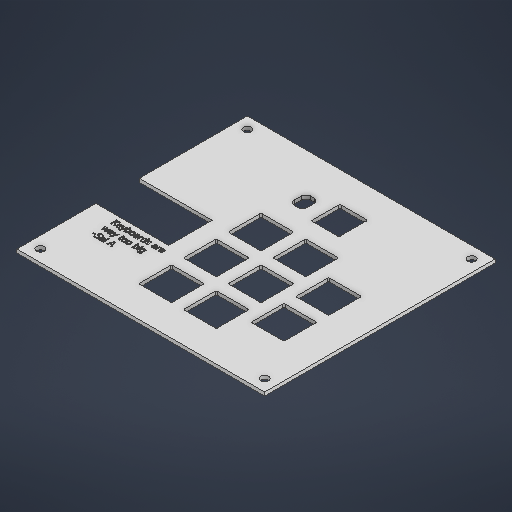
# Autodesk Inventor part: Top_Plate
Saved by Autodesk Inventor 2026 (Build 300175050, 175E)
## iProperties
Created: 2025-06-13
Part Number: Top_Plate
Material: Generic
Document SubType Name: Modeling
Designer: SaiAn
Density: 1 g/cm^3
Appearance: Default
Author: SaiAn
Autodesk Inventor part; units mm, degrees
ref_plane "YZ Plane" through (0, 0, 0) normal (1, 0, 0) x (0, 1, 0)
ref_plane "XZ Plane" through (0, 0, 0) normal (0, 1, 0) x (-1, 0, 0)
ref_plane "XY Plane" through (0, 0, 0) normal (0, 0, 1) x (1, 0, 0)
sketch "Sketch1" plane through (0, 0, 0) normal (0, 1, 0) x (-1, 0, 0)
  line L0 (0, 0) -> (105.5, 0)
  line L1 (105.5, 0) -> (105.5, -98.12)
  line L2 (105.5, -98.12) -> (0, -98.12)
  line L3 (0, -98.12) -> (0, 0)
  line L4 (34.205, -46.155) -> (47.205, -46.155)
  line L5 (33.705, -45.655) -> (33.705, -32.655)
  line L6 (47.705, -45.655) -> (47.705, -32.655)
  line L7 (34.205, -32.155) -> (47.205, -32.155)
  arc A0 (47.705, -32.655) -> (47.205, -32.155) centre (47.205, -32.655) ccw
  line L8 (34.205, -27.105) -> (47.205, -27.105)
  arc A1 (33.705, -26.605) -> (34.205, -27.105) centre (34.205, -26.605) ccw
  arc A2 (47.205, -27.105) -> (47.705, -26.605) centre (47.205, -26.605) ccw
  line L9 (33.705, -26.605) -> (33.705, -13.605)
  line L10 (47.705, -26.605) -> (47.705, -13.605)
  arc A3 (47.705, -13.605) -> (47.205, -13.105) centre (47.205, -13.605) ccw
  line L11 (34.205, -13.105) -> (47.205, -13.105)
  arc A4 (34.205, -13.105) -> (33.705, -13.605) centre (34.205, -13.605) ccw
  line L12 (33.705, -64.705) -> (33.705, -51.705)
  line L13 (47.705, -64.705) -> (47.705, -51.705)
  line L14 (34.205, -65.205) -> (47.205, -65.205)
  line L15 (34.205, -51.205) -> (47.205, -51.205)
  arc A5 (47.705, -51.705) -> (47.205, -51.205) centre (47.205, -51.705) ccw
  arc A6 (34.205, -51.205) -> (33.705, -51.705) centre (34.205, -51.705) ccw
  arc A7 (47.205, -65.205) -> (47.705, -64.705) centre (47.205, -64.705) ccw
  arc A8 (33.705, -64.705) -> (34.205, -65.205) centre (34.205, -64.705) ccw
  arc A9 (33.705, -45.655) -> (34.205, -46.155) centre (34.205, -45.655) ccw
  arc A10 (34.205, -32.155) -> (33.705, -32.655) centre (34.205, -32.655) ccw
  arc A11 (47.205, -46.155) -> (47.705, -45.655) centre (47.205, -45.655) ccw
  line L16 (52.755, -64.705) -> (52.755, -51.705)
  line L17 (66.755, -64.705) -> (66.755, -51.705)
  line L18 (53.255, -65.205) -> (66.255, -65.205)
  arc A12 (66.255, -65.205) -> (66.755, -64.705) centre (66.255, -64.705) ccw
  arc A13 (52.755, -45.655) -> (53.255, -46.155) centre (53.255, -45.655) ccw
  arc A14 (53.255, -51.205) -> (52.755, -51.705) centre (53.255, -51.705) ccw
  arc A15 (66.255, -46.155) -> (66.755, -45.655) centre (66.255, -45.655) ccw
  line L19 (53.255, -51.205) -> (66.255, -51.205)
  arc A16 (52.755, -64.705) -> (53.255, -65.205) centre (53.255, -64.705) ccw
  line L20 (53.255, -46.155) -> (66.255, -46.155)
  line L21 (66.755, -45.655) -> (66.755, -32.655)
  line L22 (53.255, -32.155) -> (66.255, -32.155)
  arc A17 (53.255, -32.155) -> (52.755, -32.655) centre (53.255, -32.655) ccw
  line L23 (52.755, -45.655) -> (52.755, -32.655)
  arc A18 (66.755, -51.705) -> (66.255, -51.205) centre (66.255, -51.705) ccw
  arc A19 (66.755, -32.655) -> (66.255, -32.155) centre (66.255, -32.655) ccw
  line L24 (53.255, -27.105) -> (66.255, -27.105)
  arc A20 (52.755, -26.605) -> (53.255, -27.105) centre (53.255, -26.605) ccw
  arc A21 (66.255, -27.105) -> (66.755, -26.605) centre (66.255, -26.605) ccw
  line L25 (52.755, -26.605) -> (52.755, -13.605)
  line L26 (53.255, -13.105) -> (66.255, -13.105)
  line L27 (66.755, -26.605) -> (66.755, -13.605)
  arc A22 (53.255, -13.105) -> (52.755, -13.605) centre (53.255, -13.605) ccw
  arc A23 (66.755, -13.605) -> (66.255, -13.105) centre (66.255, -13.605) ccw
  line L28 (14.6002, -55.3601) -> (14.6002, -42.3601)
  arc A24 (14.6002, -55.3601) -> (15.1002, -55.8601) centre (15.1002, -55.3601) ccw
  arc A25 (28.6002, -42.3601) -> (28.1002, -41.8601) centre (28.1002, -42.3601) ccw
  arc A26 (28.1002, -55.8601) -> (28.6002, -55.3601) centre (28.1002, -55.3601) ccw
  line L29 (28.6002, -55.3601) -> (28.6002, -42.3601)
  line L30 (15.1002, -55.8601) -> (28.1002, -55.8601)
  line L31 (15.1002, -41.8601) -> (28.1002, -41.8601)
  arc A27 (15.1002, -41.8601) -> (14.6002, -42.3601) centre (15.1002, -42.3601) ccw
  line L32 (15.1002, -36.8101) -> (28.1002, -36.8101)
  arc A28 (28.1002, -36.8101) -> (28.6002, -36.3101) centre (28.1002, -36.3101) ccw
  line L33 (14.6002, -36.3101) -> (14.6002, -23.3101)
  line L34 (28.6002, -36.3101) -> (28.6002, -23.3101)
  arc A29 (15.1002, -22.8101) -> (14.6002, -23.3101) centre (15.1002, -23.3101) ccw
  line L35 (15.1002, -22.8101) -> (28.1002, -22.8101)
  arc A30 (28.6002, -23.3101) -> (28.1002, -22.8101) centre (28.1002, -23.3101) ccw
  arc A31 (14.6002, -36.3101) -> (15.1002, -36.8101) centre (15.1002, -36.3101) ccw
  line L36 (62.477, -82.084) -> (60.977, -82.084)
  line L37 (58.977, -80.084) -> (58.977, -77.084)
  line L38 (60.977, -75.084) -> (62.477, -75.084)
  line L39 (64.477, -77.084) -> (64.477, -80.084)
  arc A32 (64.477, -77.084) -> (62.477, -75.084) centre (62.477, -77.084) ccw
  arc A33 (62.477, -82.084) -> (64.477, -80.084) centre (62.477, -80.084) ccw
  arc A34 (60.977, -75.084) -> (58.977, -77.084) centre (60.977, -77.084) ccw
  arc A35 (58.977, -80.084) -> (60.977, -82.084) centre (60.977, -80.084) ccw
  line L40 (105.5, -98.12) -> (105.5, -85.262)
  line L41 (52.74, -85.262) -> (41.94, -85.262)
  line L42 (41.44, -84.762) -> (41.44, -73.562)
  line L43 (41.94, -73.062) -> (52.74, -73.062)
  line L44 (53.24, -73.562) -> (53.24, -84.762)
  arc A36 (52.74, -85.262) -> (53.24, -84.762) centre (52.74, -84.762) ccw
  arc A37 (53.24, -73.562) -> (52.74, -73.062) centre (52.74, -73.562) ccw
  arc A38 (41.94, -73.062) -> (41.44, -73.562) centre (41.94, -73.562) ccw
  arc A39 (41.44, -84.762) -> (41.94, -85.262) centre (41.94, -84.762) ccw
  line L45 (105.5, -33.622) -> (74.5, -33.622)
  line L46 (74.5, -33.622) -> (74.5, -52.122)
  line L47 (74.5, -52.122) -> (105.5, -52.122)
  line L48 (105.5, -33.622) -> (105.5, -52.122)
  circle A40 centre (100.5, -5) radius 1.7
  circle A41 centre (100.5, -93.12) radius 1.7
  circle A42 centre (5, -5) radius 1.7
  circle A43 centre (5, -93.12) radius 1.7
  point P0 (53.24, -85.262)
  point P1 (41.44, -73.062)
  point P2 (41.44, -85.262)
  point P3 (53.24, -73.062)
  point P4 (15.1002, -22.8101)
  point P5 (28.6002, -36.3101)
  point P6 (15.1002, -55.8601)
  point P7 (28.1002, -41.8601)
  point P8 (28.6002, -42.3601)
  point P9 (28.6002, -55.3601)
  point P10 (28.1002, -55.8601)
  point P11 (66.755, -26.605)
  point P12 (66.755, -45.655)
  point P13 (66.255, -46.155)
  point P14 (53.255, -46.155)
  point P15 (52.755, -45.655)
  point P16 (52.755, -32.655)
  point P17 (53.255, -51.205)
  point P18 (33.705, -26.605)
  point P19 (47.205, -13.105)
  point P20 (47.705, -26.605)
  dimension "d0" = 105.5
  dimension "d1" = 98.12
  dimension "d16" = 2
  dimension "d17" = 2
  dimension "d18" = 2
  dimension "d19" = 2
  dimension "d21" = 52.26
  dimension "d22" = 11.8
  dimension "d23" = 12.2
  dimension "d24" = 0.5
  dimension "d26" = 31
  dimension "d28" = 18.5
  dimension "d29" = 3.4
  dimension "d30" = 3.4
  dimension "d31" = 3.4
  dimension "d32" = 3.4
  dimension "d33" = 5
  dimension "d34" = 5
  dimension "d35" = 5
  dimension "d36" = 5
  dimension "d37" = 5
  dimension "d38" = 5
  dimension "d39" = 5
  dimension "d40" = 5
  constraints: 98 end point, 80 point on circle, 44 centre point, 16 tangent, 11 point on line, 6 parallel, 5 perpendicular, 3 equal radius, 3 horizontal, 1 collinear
  measures "d0" distance of L1.end L2.end
  measures "d1" distance of L0.end L1.end
  measures "d16" radius of A32
  measures "d17" radius of A33
  measures "d18" radius of A34
  measures "d19" radius of A35
  measures "d21" distance of L40.end point (53.24, -85.262)
  measures "d22" distance of point (41.44, -73.062) point (53.24, -73.062)
  measures "d23" distance of point (41.44, -85.262) point (41.44, -73.062)
  measures "d24" radius of A36
  measures "d26" distance of L45.start L45.end
  measures "d28" distance of L45.end L46.end
  measures "d29" diameter of A40
  measures "d30" diameter of A41
  measures "d31" diameter of A42
  measures "d32" diameter of A43
  measures "d33" distance from line of L1 A40.centre
  measures "d34" distance from line of L0 A40.centre
  measures "d35" distance from line of L2 A41.centre
  measures "d36" distance from line of L1 A41.centre
  measures "d37" distance from line of L0 A42.centre
  measures "d38" distance from line of L3 A42.centre
  measures "d39" distance from line of L2 A43.centre
  measures "d40" distance from line of L3 A43.centre
extrude "Extrusion1" add sketch "Sketch1" along normal blind 1.5 contours L0 L1 L45 L46 L47 L2 L3
sketch "Sketch3" plane through (0, 1.5, 0) normal (0, 1, 0) x (1, 0, 0)
  line L0 (-95.2585, 32.0285) -> (-71.0604, 32.0285) construction
  line L1 (-71.0604, 32.0285) -> (-71.0604, 1.6863) construction
  line L2 (-71.0604, 1.6863) -> (-95.2585, 1.6863) construction
  line L3 (-95.2585, 1.6863) -> (-95.2585, 32.0285) construction
  line L4 (-93.1487, 29.3753) -> (-93.5871, 29.3753)
  line L5 (-93.5871, 29.3753) -> (-94.5154, 30.5567)
  line L6 (-94.5154, 30.5567) -> (-94.6636, 30.39)
  line L7 (-94.6636, 30.39) -> (-94.6636, 29.3753)
  line L8 (-94.6636, 29.3753) -> (-95.0012, 29.3753)
  line L9 (-95.0012, 29.3753) -> (-95.0012, 31.9153)
  line L10 (-95.0012, 31.9153) -> (-94.6636, 31.9153)
  line L11 (-94.6636, 31.9153) -> (-94.6636, 30.7482)
  line L12 (-94.6636, 30.7482) -> (-93.6221, 31.9153)
  line L13 (-93.6221, 31.9153) -> (-93.2104, 31.9153)
  line L14 (-93.2104, 31.9153) -> (-94.2623, 30.7811)
  line L15 (-94.2623, 30.7811) -> (-93.1487, 29.3753)
  spline S0 degree 2 poles (-92.1442, 29.332) (-92.6012, 29.332) (-93.1034, 29.8446) (-93.1034, 30.318) knots 0 0 0 1 2 2 2
  spline S1 degree 2 poles (-93.1034, 30.318) (-93.1034, 30.7832) (-92.6156, 31.3348) (-92.2224, 31.3348) knots 0 0 0 1 2 2 2
  spline S2 degree 2 poles (-92.2224, 31.3348) (-92.0454, 31.3348) (-91.7717, 31.2319) (-91.6708, 31.1228) knots 0 0 0 1 2 2 2
  spline S3 degree 2 poles (-91.6708, 31.1228) (-91.5679, 31.0137) (-91.4588, 30.6988) (-91.4588, 30.4703) knots 0 0 0 1 2 2 2
  line L16 (-91.4588, 30.4703) -> (-91.4588, 30.2953)
  line L17 (-91.4588, 30.2953) -> (-92.7782, 30.2953)
  spline S4 degree 2 poles (-92.7782, 30.2953) (-92.7782, 29.9639) (-92.4447, 29.612) (-92.1483, 29.612) knots 0 0 0 1 2 2 2
  spline S5 degree 2 poles (-92.1483, 29.612) (-92.0434, 29.612) (-91.8396, 29.6593) (-91.7572, 29.6964) knots 0 0 0 1 2 2 2
  spline S6 degree 2 poles (-91.7572, 29.6964) (-91.6708, 29.7375) (-91.5514, 29.8096) (-91.5123, 29.8425) knots 0 0 0 1 2 2 2
  line L18 (-91.5123, 29.8425) -> (-91.4938, 29.8425)
  line L19 (-91.4938, 29.8425) -> (-91.4938, 29.4926)
  spline S7 degree 2 poles (-91.4938, 29.4926) (-91.5494, 29.4699) (-91.7181, 29.4041) (-91.784, 29.3855) knots 0 0 0 1 2 2 2
  spline S8 degree 2 poles (-91.784, 29.3855) (-91.8766, 29.3588) (-92.0289, 29.332) (-92.1442, 29.332) knots 0 0 0 1 2 2 2
  spline S9 degree 2 poles (-91.7717, 30.5403) (-91.7758, 30.67) (-91.8293, 30.8593) (-91.8807, 30.9231) knots 0 0 0 1 2 2 2
  spline S10 degree 2 poles (-91.8807, 30.9231) (-91.9363, 30.9952) (-92.1113, 31.0713) (-92.241, 31.0713) knots 0 0 0 1 2 2 2
  spline S11 degree 2 poles (-92.241, 31.0713) (-92.3686, 31.0713) (-92.5476, 30.9952) (-92.6217, 30.9211) knots 0 0 0 1 2 2 2
  spline S12 degree 2 poles (-92.6217, 30.9211) (-92.6938, 30.8449) (-92.7679, 30.6617) (-92.7782, 30.5403) knots 0 0 0 1 2 2 2
  line L20 (-92.7782, 30.5403) -> (-91.7717, 30.5403)
  line L21 (-89.6371, 31.2813) -> (-90.6622, 28.6734)
  line L22 (-90.6622, 28.6734) -> (-91.0059, 28.6734)
  line L23 (-91.0059, 28.6734) -> (-90.6643, 29.4679)
  line L24 (-90.6643, 29.4679) -> (-91.3559, 31.2813)
  line L25 (-91.3559, 31.2813) -> (-91.0101, 31.2813)
  line L26 (-91.0101, 31.2813) -> (-90.4893, 29.8693)
  line L27 (-90.4893, 29.8693) -> (-89.9706, 31.2813)
  line L28 (-89.9706, 31.2813) -> (-89.6371, 31.2813)
  spline S13 degree 2 poles (-87.797, 30.3591) (-87.797, 29.8919) (-88.2498, 29.3217) (-88.5915, 29.3217) knots 0 0 0 1 2 2 2
  spline S14 degree 2 poles (-88.5915, 29.3217) (-88.7459, 29.3217) (-88.9661, 29.3979) (-89.0732, 29.4638) knots 0 0 0 1 2 2 2
  line L29 (-89.0732, 29.4638) -> (-89.0937, 29.3753)
  line L30 (-89.0937, 29.3753) -> (-89.3943, 29.3753)
  line L31 (-89.3943, 29.3753) -> (-89.3943, 32.0285)
  line L32 (-89.3943, 32.0285) -> (-89.0732, 32.0285)
  line L33 (-89.0732, 32.0285) -> (-89.0732, 31.0816)
  spline S15 degree 2 poles (-89.0732, 31.0816) (-88.9517, 31.1907) (-88.6697, 31.3348) (-88.4906, 31.3348) knots 0 0 0 1 2 2 2
  spline S16 degree 2 poles (-88.4906, 31.3348) (-88.1675, 31.3348) (-87.797, 30.8182) (-87.797, 30.3591) knots 0 0 0 1 2 2 2
  spline S17 degree 2 poles (-88.1284, 30.3344) (-88.1284, 30.6761) (-88.3363, 31.0302) (-88.5668, 31.0302) knots 0 0 0 1 2 2 2
  spline S18 degree 2 poles (-88.5668, 31.0302) (-88.6965, 31.0302) (-88.9641, 30.9067) (-89.0732, 30.812) knots 0 0 0 1 2 2 2
  line L34 (-89.0732, 30.812) -> (-89.0732, 29.719)
  spline S19 degree 2 poles (-89.0732, 29.719) (-88.9517, 29.6593) (-88.7644, 29.6099) (-88.6533, 29.6099) knots 0 0 0 1 2 2 2
  spline S20 degree 2 poles (-88.6533, 29.6099) (-88.4083, 29.6099) (-88.1284, 29.9578) (-88.1284, 30.3344) knots 0 0 0 1 2 2 2
  spline S21 degree 2 poles (-85.8971, 30.3283) (-85.8971, 29.8466) (-86.3603, 29.3217) (-86.7472, 29.3217) knots 0 0 0 1 2 2 2
  spline S22 degree 2 poles (-86.7472, 29.3217) (-87.1445, 29.3217) (-87.5994, 29.8631) (-87.5994, 30.3283) knots 0 0 0 1 2 2 2
  spline S23 degree 2 poles (-87.5994, 30.3283) (-87.5994, 30.8058) (-87.1301, 31.3348) (-86.7472, 31.3348) knots 0 0 0 1 2 2 2
  spline S24 degree 2 poles (-86.7472, 31.3348) (-86.3603, 31.3348) (-85.8971, 30.8079) (-85.8971, 30.3283) knots 0 0 0 1 2 2 2
  spline S25 degree 2 poles (-86.2285, 30.3283) (-86.2285, 30.6988) (-86.4982, 31.059) (-86.7472, 31.059) knots 0 0 0 1 2 2 2
  spline S26 degree 2 poles (-86.7472, 31.059) (-86.9963, 31.059) (-87.268, 30.6988) (-87.268, 30.3283) knots 0 0 0 1 2 2 2
  spline S27 degree 2 poles (-87.268, 30.3283) (-87.268, 29.9681) (-86.9963, 29.5976) (-86.7472, 29.5976) knots 0 0 0 1 2 2 2
  spline S28 degree 2 poles (-86.7472, 29.5976) (-86.5002, 29.5976) (-86.2285, 29.9619) (-86.2285, 30.3283) knots 0 0 0 1 2 2 2
  spline S29 degree 2 poles (-84.5057, 29.577) (-84.5448, 29.5482) (-84.6765, 29.4452) (-84.7383, 29.4144) knots 0 0 0 1 2 2 2
  spline S30 degree 2 poles (-84.7383, 29.4144) (-84.8227, 29.3691) (-84.9812, 29.3217) (-85.1252, 29.3217) knots 0 0 0 1 2 2 2
  spline S31 degree 2 poles (-85.1252, 29.3217) (-85.2426, 29.3217) (-85.4546, 29.4102) (-85.5349, 29.4905) knots 0 0 0 1 2 2 2
  spline S32 degree 2 poles (-85.5349, 29.4905) (-85.611, 29.5687) (-85.7036, 29.7993) (-85.7036, 29.9269) knots 0 0 0 1 2 2 2
  spline S33 degree 2 poles (-85.7036, 29.9269) (-85.7036, 30.1245) (-85.5369, 30.4044) (-85.3558, 30.4847) knots 0 0 0 1 2 2 2
  spline S34 degree 2 poles (-85.3558, 30.4847) (-85.1952, 30.5588) (-84.7589, 30.6144) (-84.5057, 30.6288) knots 0 0 0 1 2 2 2
  line L35 (-84.5057, 30.6288) -> (-84.5057, 30.6905)
  spline S35 degree 2 poles (-84.5057, 30.6905) (-84.5057, 30.8017) (-84.5736, 30.9396) (-84.6354, 30.9787) knots 0 0 0 1 2 2 2
  spline S36 degree 2 poles (-84.6354, 30.9787) (-84.6971, 31.0178) (-84.8741, 31.0425) (-84.9688, 31.0425) knots 0 0 0 1 2 2 2
  spline S37 degree 2 poles (-84.9688, 31.0425) (-85.08, 31.0425) (-85.3805, 30.9766) (-85.5307, 30.9128) knots 0 0 0 1 2 2 2
  line L36 (-85.5307, 30.9128) -> (-85.5493, 30.9128)
  line L37 (-85.5493, 30.9128) -> (-85.5493, 31.2401)
  spline S38 degree 2 poles (-85.5493, 31.2401) (-85.4608, 31.2648) (-85.1294, 31.3266) (-84.9668, 31.3266) knots 0 0 0 1 2 2 2
  spline S39 degree 2 poles (-84.9668, 31.3266) (-84.7692, 31.3266) (-84.4995, 31.2648) (-84.3925, 31.1845) knots 0 0 0 1 2 2 2
  spline S40 degree 2 poles (-84.3925, 31.1845) (-84.2875, 31.1063) (-84.1846, 30.8573) (-84.1846, 30.6782) knots 0 0 0 1 2 2 2
  line L38 (-84.1846, 30.6782) -> (-84.1846, 29.3753)
  line L39 (-84.1846, 29.3753) -> (-84.5057, 29.3753)
  line L40 (-84.5057, 29.3753) -> (-84.5057, 29.577)
  line L41 (-84.5057, 29.8446) -> (-84.5057, 30.3736)
  spline S41 degree 2 poles (-84.5057, 30.3736) (-84.621, 30.3633) (-84.9688, 30.3283) (-85.0779, 30.2953) knots 0 0 0 1 2 2 2
  spline S42 degree 2 poles (-85.0779, 30.2953) (-85.2055, 30.2562) (-85.3723, 30.0936) (-85.3723, 29.9495) knots 0 0 0 1 2 2 2
  spline S43 degree 2 poles (-85.3723, 29.9495) (-85.3723, 29.7849) (-85.187, 29.6181) (-85.01, 29.6181) knots 0 0 0 1 2 2 2
  spline S44 degree 2 poles (-85.01, 29.6181) (-84.8597, 29.6181) (-84.6127, 29.7478) (-84.5057, 29.8446) knots 0 0 0 1 2 2 2
  line L42 (-82.7232, 30.9375) -> (-82.7396, 30.9375)
  spline S45 degree 2 poles (-82.7396, 30.9375) (-82.7767, 30.9478) (-82.857, 30.9519) (-82.9125, 30.9519) knots 0 0 0 1 2 2 2
  spline S46 degree 2 poles (-82.9125, 30.9519) (-83.0422, 30.9519) (-83.2974, 30.8387) (-83.4127, 30.7276) knots 0 0 0 1 2 2 2
  line L43 (-83.4127, 30.7276) -> (-83.4127, 29.3753)
  line L44 (-83.4127, 29.3753) -> (-83.7338, 29.3753)
  line L45 (-83.7338, 29.3753) -> (-83.7338, 31.2813)
  line L46 (-83.7338, 31.2813) -> (-83.4127, 31.2813)
  line L47 (-83.4127, 31.2813) -> (-83.4127, 30.9972)
  spline S47 degree 2 poles (-83.4127, 30.9972) (-83.2377, 31.1537) (-82.9763, 31.2813) (-82.8528, 31.2813) knots 0 0 0 1 2 2 2
  spline S48 degree 2 poles (-82.8528, 31.2813) (-82.8034, 31.2813) (-82.754, 31.2772) (-82.7232, 31.271) knots 0 0 0 1 2 2 2
  line L48 (-82.7232, 31.271) -> (-82.7232, 30.9375)
  line L49 (-81.0086, 29.3753) -> (-81.3297, 29.3753)
  line L50 (-81.3297, 29.3753) -> (-81.3297, 29.5687)
  spline S49 degree 2 poles (-81.3297, 29.5687) (-81.4038, 29.507) (-81.5129, 29.4247) (-81.587, 29.3897) knots 0 0 0 1 2 2 2
  spline S50 degree 2 poles (-81.587, 29.3897) (-81.6549, 29.3567) (-81.801, 29.3217) (-81.8978, 29.3217) knots 0 0 0 1 2 2 2
  spline S51 degree 2 poles (-81.8978, 29.3217) (-82.0542, 29.3217) (-82.3177, 29.4514) (-82.4103, 29.577) knots 0 0 0 1 2 2 2
  spline S52 degree 2 poles (-82.4103, 29.577) (-82.5029, 29.7025) (-82.6058, 30.073) (-82.6058, 30.3139) knots 0 0 0 1 2 2 2
  spline S53 degree 2 poles (-82.6058, 30.3139) (-82.6058, 30.565) (-82.4762, 30.9314) (-82.3629, 31.0693) knots 0 0 0 1 2 2 2
  spline S54 degree 2 poles (-82.3629, 31.0693) (-82.258, 31.1928) (-81.9636, 31.3348) (-81.801, 31.3348) knots 0 0 0 1 2 2 2
  spline S55 degree 2 poles (-81.801, 31.3348) (-81.659, 31.3348) (-81.447, 31.271) (-81.3297, 31.2051) knots 0 0 0 1 2 2 2
  line L51 (-81.3297, 31.2051) -> (-81.3297, 32.0285)
  line L52 (-81.3297, 32.0285) -> (-81.0086, 32.0285)
  line L53 (-81.0086, 32.0285) -> (-81.0086, 29.3753)
  line L54 (-81.3297, 29.8384) -> (-81.3297, 30.9396)
  spline S56 degree 2 poles (-81.3297, 30.9396) (-81.449, 30.9972) (-81.6384, 31.0405) (-81.7475, 31.0405) knots 0 0 0 1 2 2 2
  spline S57 degree 2 poles (-81.7475, 31.0405) (-81.9945, 31.0405) (-82.2744, 30.67) (-82.2744, 30.32) knots 0 0 0 1 2 2 2
  spline S58 degree 2 poles (-82.2744, 30.32) (-82.2744, 29.9825) (-82.0604, 29.6264) (-81.8237, 29.6264) knots 0 0 0 1 2 2 2
  spline S59 degree 2 poles (-81.8237, 29.6264) (-81.6981, 29.6264) (-81.4429, 29.7416) (-81.3297, 29.8384) knots 0 0 0 1 2 2 2
  spline S60 degree 2 poles (-80.0288, 29.33) (-80.2202, 29.33) (-80.5516, 29.4329) (-80.6607, 29.4905) knots 0 0 0 1 2 2 2
  line L55 (-80.6607, 29.4905) -> (-80.6607, 29.8507)
  line L56 (-80.6607, 29.8507) -> (-80.6442, 29.8507)
  spline S61 degree 2 poles (-80.6442, 29.8507) (-80.6031, 29.8178) (-80.4919, 29.7396) (-80.3993, 29.6964) knots 0 0 0 1 2 2 2
  spline S62 degree 2 poles (-80.3993, 29.6964) (-80.319, 29.6572) (-80.1214, 29.5996) (-80.0164, 29.5996) knots 0 0 0 1 2 2 2
  spline S63 degree 2 poles (-80.0164, 29.5996) (-79.9403, 29.5996) (-79.7653, 29.6346) (-79.7241, 29.6634) knots 0 0 0 1 2 2 2
  spline S64 degree 2 poles (-79.7241, 29.6634) (-79.6645, 29.7025) (-79.6109, 29.791) (-79.6109, 29.8816) knots 0 0 0 1 2 2 2
  spline S65 degree 2 poles (-79.6109, 29.8816) (-79.6109, 29.9948) (-79.7344, 30.1121) (-79.8929, 30.1513) knots 0 0 0 1 2 2 2
  spline S66 degree 2 poles (-79.8929, 30.1513) (-79.9547, 30.1657) (-80.1523, 30.2068) (-80.2367, 30.2295) knots 0 0 0 1 2 2 2
  spline S67 degree 2 poles (-80.2367, 30.2295) (-80.4549, 30.2933) (-80.6525, 30.5567) (-80.6525, 30.7441) knots 0 0 0 1 2 2 2
  spline S68 degree 2 poles (-80.6525, 30.7441) (-80.6525, 31.0034) (-80.2634, 31.3266) (-79.9423, 31.3266) knots 0 0 0 1 2 2 2
  spline S69 degree 2 poles (-79.9423, 31.3266) (-79.7838, 31.3266) (-79.4627, 31.2483) (-79.3536, 31.1887) knots 0 0 0 1 2 2 2
  line L57 (-79.3536, 31.1887) -> (-79.3536, 30.8449)
  line L58 (-79.3536, 30.8449) -> (-79.3701, 30.8449)
  spline S70 degree 2 poles (-79.3701, 30.8449) (-79.4936, 30.9437) (-79.7941, 31.0569) (-79.9485, 31.0569) knots 0 0 0 1 2 2 2
  spline S71 degree 2 poles (-79.9485, 31.0569) (-80.107, 31.0569) (-80.3252, 30.9231) (-80.3252, 30.7893) knots 0 0 0 1 2 2 2
  spline S72 degree 2 poles (-80.3252, 30.7893) (-80.3252, 30.6679) (-80.1955, 30.5506) (-80.0514, 30.5135) knots 0 0 0 1 2 2 2
  spline S73 degree 2 poles (-80.0514, 30.5135) (-79.9814, 30.495) (-79.8044, 30.4579) (-79.7077, 30.4353) knots 0 0 0 1 2 2 2
  spline S74 degree 2 poles (-79.7077, 30.4353) (-79.4977, 30.3818) (-79.2837, 30.1368) (-79.2837, 29.9248) knots 0 0 0 1 2 2 2
  spline S75 degree 2 poles (-79.2837, 29.9248) (-79.2837, 29.8013) (-79.3804, 29.5831) (-79.4751, 29.5029) knots 0 0 0 1 2 2 2
  spline S76 degree 2 poles (-79.4751, 29.5029) (-79.5759, 29.4185) (-79.8332, 29.33) (-80.0288, 29.33) knots 0 0 0 1 2 2 2
  spline S77 degree 2 poles (-76.8322, 29.577) (-76.8713, 29.5482) (-77.003, 29.4452) (-77.0648, 29.4144) knots 0 0 0 1 2 2 2
  spline S78 degree 2 poles (-77.0648, 29.4144) (-77.1492, 29.3691) (-77.3076, 29.3217) (-77.4517, 29.3217) knots 0 0 0 1 2 2 2
  spline S79 degree 2 poles (-77.4517, 29.3217) (-77.5691, 29.3217) (-77.7811, 29.4102) (-77.8613, 29.4905) knots 0 0 0 1 2 2 2
  spline S80 degree 2 poles (-77.8613, 29.4905) (-77.9375, 29.5687) (-78.0301, 29.7993) (-78.0301, 29.9269) knots 0 0 0 1 2 2 2
  spline S81 degree 2 poles (-78.0301, 29.9269) (-78.0301, 30.1245) (-77.8634, 30.4044) (-77.6823, 30.4847) knots 0 0 0 1 2 2 2
  spline S82 degree 2 poles (-77.6823, 30.4847) (-77.5217, 30.5588) (-77.0853, 30.6144) (-76.8322, 30.6288) knots 0 0 0 1 2 2 2
  line L59 (-76.8322, 30.6288) -> (-76.8322, 30.6905)
  spline S83 degree 2 poles (-76.8322, 30.6905) (-76.8322, 30.8017) (-76.9001, 30.9396) (-76.9618, 30.9787) knots 0 0 0 1 2 2 2
  spline S84 degree 2 poles (-76.9618, 30.9787) (-77.0236, 31.0178) (-77.2006, 31.0425) (-77.2953, 31.0425) knots 0 0 0 1 2 2 2
  spline S85 degree 2 poles (-77.2953, 31.0425) (-77.4064, 31.0425) (-77.707, 30.9766) (-77.8572, 30.9128) knots 0 0 0 1 2 2 2
  line L60 (-77.8572, 30.9128) -> (-77.8758, 30.9128)
  line L61 (-77.8758, 30.9128) -> (-77.8758, 31.2401)
  spline S86 degree 2 poles (-77.8758, 31.2401) (-77.7872, 31.2648) (-77.4558, 31.3266) (-77.2932, 31.3266) knots 0 0 0 1 2 2 2
  spline S87 degree 2 poles (-77.2932, 31.3266) (-77.0956, 31.3266) (-76.826, 31.2648) (-76.719, 31.1845) knots 0 0 0 1 2 2 2
  spline S88 degree 2 poles (-76.719, 31.1845) (-76.614, 31.1063) (-76.5111, 30.8573) (-76.5111, 30.6782) knots 0 0 0 1 2 2 2
  line L62 (-76.5111, 30.6782) -> (-76.5111, 29.3753)
  line L63 (-76.5111, 29.3753) -> (-76.8322, 29.3753)
  line L64 (-76.8322, 29.3753) -> (-76.8322, 29.577)
  line L65 (-76.8322, 29.8446) -> (-76.8322, 30.3736)
  spline S89 degree 2 poles (-76.8322, 30.3736) (-76.9474, 30.3633) (-77.2953, 30.3283) (-77.4044, 30.2953) knots 0 0 0 1 2 2 2
  spline S90 degree 2 poles (-77.4044, 30.2953) (-77.532, 30.2562) (-77.6987, 30.0936) (-77.6987, 29.9495) knots 0 0 0 1 2 2 2
  spline S91 degree 2 poles (-77.6987, 29.9495) (-77.6987, 29.7849) (-77.5135, 29.6181) (-77.3365, 29.6181) knots 0 0 0 1 2 2 2
  spline S92 degree 2 poles (-77.3365, 29.6181) (-77.1862, 29.6181) (-76.9392, 29.7478) (-76.8322, 29.8446) knots 0 0 0 1 2 2 2
  line L66 (-75.0496, 30.9375) -> (-75.0661, 30.9375)
  spline S93 degree 2 poles (-75.0661, 30.9375) (-75.1032, 30.9478) (-75.1834, 30.9519) (-75.239, 30.9519) knots 0 0 0 1 2 2 2
  spline S94 degree 2 poles (-75.239, 30.9519) (-75.3687, 30.9519) (-75.6239, 30.8387) (-75.7392, 30.7276) knots 0 0 0 1 2 2 2
  line L67 (-75.7392, 30.7276) -> (-75.7392, 29.3753)
  line L68 (-75.7392, 29.3753) -> (-76.0603, 29.3753)
  line L69 (-76.0603, 29.3753) -> (-76.0603, 31.2813)
  line L70 (-76.0603, 31.2813) -> (-75.7392, 31.2813)
  line L71 (-75.7392, 31.2813) -> (-75.7392, 30.9972)
  spline S95 degree 2 poles (-75.7392, 30.9972) (-75.5642, 31.1537) (-75.3028, 31.2813) (-75.1793, 31.2813) knots 0 0 0 1 2 2 2
  spline S96 degree 2 poles (-75.1793, 31.2813) (-75.1299, 31.2813) (-75.0805, 31.2772) (-75.0496, 31.271) knots 0 0 0 1 2 2 2
  line L72 (-75.0496, 31.271) -> (-75.0496, 30.9375)
  spline S97 degree 2 poles (-73.9731, 29.332) (-74.4301, 29.332) (-74.9323, 29.8446) (-74.9323, 30.318) knots 0 0 0 1 2 2 2
  spline S98 degree 2 poles (-74.9323, 30.318) (-74.9323, 30.7832) (-74.4445, 31.3348) (-74.0513, 31.3348) knots 0 0 0 1 2 2 2
  spline S99 degree 2 poles (-74.0513, 31.3348) (-73.8743, 31.3348) (-73.6006, 31.2319) (-73.4997, 31.1228) knots 0 0 0 1 2 2 2
  spline S100 degree 2 poles (-73.4997, 31.1228) (-73.3968, 31.0137) (-73.2877, 30.6988) (-73.2877, 30.4703) knots 0 0 0 1 2 2 2
  line L73 (-73.2877, 30.4703) -> (-73.2877, 30.2953)
  line L74 (-73.2877, 30.2953) -> (-74.6071, 30.2953)
  spline S101 degree 2 poles (-74.6071, 30.2953) (-74.6071, 29.9639) (-74.2736, 29.612) (-73.9772, 29.612) knots 0 0 0 1 2 2 2
  spline S102 degree 2 poles (-73.9772, 29.612) (-73.8723, 29.612) (-73.6685, 29.6593) (-73.5862, 29.6964) knots 0 0 0 1 2 2 2
  spline S103 degree 2 poles (-73.5862, 29.6964) (-73.4997, 29.7375) (-73.3803, 29.8096) (-73.3412, 29.8425) knots 0 0 0 1 2 2 2
  line L75 (-73.3412, 29.8425) -> (-73.3227, 29.8425)
  line L76 (-73.3227, 29.8425) -> (-73.3227, 29.4926)
  spline S104 degree 2 poles (-73.3227, 29.4926) (-73.3783, 29.4699) (-73.547, 29.4041) (-73.6129, 29.3855) knots 0 0 0 1 2 2 2
  spline S105 degree 2 poles (-73.6129, 29.3855) (-73.7055, 29.3588) (-73.8579, 29.332) (-73.9731, 29.332) knots 0 0 0 1 2 2 2
  spline S106 degree 2 poles (-73.6006, 30.5403) (-73.6047, 30.67) (-73.6582, 30.8593) (-73.7097, 30.9231) knots 0 0 0 1 2 2 2
  spline S107 degree 2 poles (-73.7097, 30.9231) (-73.7652, 30.9952) (-73.9402, 31.0713) (-74.0699, 31.0713) knots 0 0 0 1 2 2 2
  spline S108 degree 2 poles (-74.0699, 31.0713) (-74.1975, 31.0713) (-74.3766, 30.9952) (-74.4507, 30.9211) knots 0 0 0 1 2 2 2
  spline S109 degree 2 poles (-74.4507, 30.9211) (-74.5227, 30.8449) (-74.5968, 30.6617) (-74.6071, 30.5403) knots 0 0 0 1 2 2 2
  line L77 (-74.6071, 30.5403) -> (-73.6006, 30.5403)
  line L78 (-92.7164, 27.0992) -> (-93.2001, 25.1932)
  line L79 (-93.2001, 25.1932) -> (-93.4965, 25.1932)
  line L80 (-93.4965, 25.1932) -> (-93.9617, 26.6629)
  line L81 (-93.9617, 26.6629) -> (-94.4249, 25.1932)
  line L82 (-94.4249, 25.1932) -> (-94.7192, 25.1932)
  line L83 (-94.7192, 25.1932) -> (-95.207, 27.0992)
  line L84 (-95.207, 27.0992) -> (-94.8736, 27.0992)
  line L85 (-94.8736, 27.0992) -> (-94.536, 25.6234)
  line L86 (-94.536, 25.6234) -> (-94.0852, 27.0992)
  line L87 (-94.0852, 27.0992) -> (-93.8197, 27.0992)
  line L88 (-93.8197, 27.0992) -> (-93.3566, 25.6234)
  line L89 (-93.3566, 25.6234) -> (-93.0396, 27.0992)
  line L90 (-93.0396, 27.0992) -> (-92.7164, 27.0992)
  spline S110 degree 2 poles (-91.3723, 25.3949) (-91.4114, 25.3661) (-91.5432, 25.2632) (-91.6049, 25.2323) knots 0 0 0 1 2 2 2
  spline S111 degree 2 poles (-91.6049, 25.2323) (-91.6893, 25.187) (-91.8478, 25.1397) (-91.9919, 25.1397) knots 0 0 0 1 2 2 2
  spline S112 degree 2 poles (-91.9919, 25.1397) (-92.1092, 25.1397) (-92.3212, 25.2282) (-92.4015, 25.3085) knots 0 0 0 1 2 2 2
  spline S113 degree 2 poles (-92.4015, 25.3085) (-92.4777, 25.3867) (-92.5703, 25.6172) (-92.5703, 25.7448) knots 0 0 0 1 2 2 2
  spline S114 degree 2 poles (-92.5703, 25.7448) (-92.5703, 25.9424) (-92.4036, 26.2224) (-92.2224, 26.3027) knots 0 0 0 1 2 2 2
  spline S115 degree 2 poles (-92.2224, 26.3027) (-92.0619, 26.3768) (-91.6255, 26.4323) (-91.3723, 26.4467) knots 0 0 0 1 2 2 2
  line L91 (-91.3723, 26.4467) -> (-91.3723, 26.5085)
  spline S116 degree 2 poles (-91.3723, 26.5085) (-91.3723, 26.6196) (-91.4403, 26.7576) (-91.502, 26.7967) knots 0 0 0 1 2 2 2
  spline S117 degree 2 poles (-91.502, 26.7967) (-91.5638, 26.8358) (-91.7408, 26.8605) (-91.8355, 26.8605) knots 0 0 0 1 2 2 2
  spline S118 degree 2 poles (-91.8355, 26.8605) (-91.9466, 26.8605) (-92.2471, 26.7946) (-92.3974, 26.7308) knots 0 0 0 1 2 2 2
  line L92 (-92.3974, 26.7308) -> (-92.4159, 26.7308)
  line L93 (-92.4159, 26.7308) -> (-92.4159, 27.0581)
  spline S119 degree 2 poles (-92.4159, 27.0581) (-92.3274, 27.0828) (-91.996, 27.1445) (-91.8334, 27.1445) knots 0 0 0 1 2 2 2
  spline S120 degree 2 poles (-91.8334, 27.1445) (-91.6358, 27.1445) (-91.3662, 27.0828) (-91.2591, 27.0025) knots 0 0 0 1 2 2 2
  spline S121 degree 2 poles (-91.2591, 27.0025) (-91.1541, 26.9243) (-91.0512, 26.6752) (-91.0512, 26.4961) knots 0 0 0 1 2 2 2
  line L94 (-91.0512, 26.4961) -> (-91.0512, 25.1932)
  line L95 (-91.0512, 25.1932) -> (-91.3723, 25.1932)
  line L96 (-91.3723, 25.1932) -> (-91.3723, 25.3949)
  line L97 (-91.3723, 25.6625) -> (-91.3723, 26.1915)
  spline S122 degree 2 poles (-91.3723, 26.1915) (-91.4876, 26.1812) (-91.8355, 26.1462) (-91.9446, 26.1133) knots 0 0 0 1 2 2 2
  spline S123 degree 2 poles (-91.9446, 26.1133) (-92.0722, 26.0742) (-92.2389, 25.9116) (-92.2389, 25.7675) knots 0 0 0 1 2 2 2
  spline S124 degree 2 poles (-92.2389, 25.7675) (-92.2389, 25.6028) (-92.0536, 25.4361) (-91.8766, 25.4361) knots 0 0 0 1 2 2 2
  spline S125 degree 2 poles (-91.8766, 25.4361) (-91.7264, 25.4361) (-91.4794, 25.5658) (-91.3723, 25.6625) knots 0 0 0 1 2 2 2
  line L98 (-89.104, 27.0992) -> (-90.1291, 24.4913)
  line L99 (-90.1291, 24.4913) -> (-90.4728, 24.4913)
  line L100 (-90.4728, 24.4913) -> (-90.1311, 25.2858)
  line L101 (-90.1311, 25.2858) -> (-90.8228, 27.0992)
  line L102 (-90.8228, 27.0992) -> (-90.477, 27.0992)
  line L103 (-90.477, 27.0992) -> (-89.9562, 25.6872)
  line L104 (-89.9562, 25.6872) -> (-89.4375, 27.0992)
  line L105 (-89.4375, 27.0992) -> (-89.104, 27.0992)
  spline S126 degree 2 poles (-87.1939, 25.1562) (-87.4553, 25.1562) (-87.7496, 25.4546) (-87.7496, 25.7778) knots 0 0 0 1 2 2 2
  line L106 (-87.7496, 25.7778) -> (-87.7496, 26.8337)
  line L107 (-87.7496, 26.8337) -> (-87.9658, 26.8337)
  line L108 (-87.9658, 26.8337) -> (-87.9658, 27.0992)
  line L109 (-87.9658, 27.0992) -> (-87.7496, 27.0992)
  line L110 (-87.7496, 27.0992) -> (-87.7496, 27.6468)
  line L111 (-87.7496, 27.6468) -> (-87.4285, 27.6468)
  line L112 (-87.4285, 27.6468) -> (-87.4285, 27.0992)
  line L113 (-87.4285, 27.0992) -> (-86.8378, 27.0992)
  line L114 (-86.8378, 27.0992) -> (-86.8378, 26.8337)
  line L115 (-86.8378, 26.8337) -> (-87.4285, 26.8337)
  line L116 (-87.4285, 26.8337) -> (-87.4285, 25.926)
  spline S127 degree 2 poles (-87.4285, 25.926) (-87.4285, 25.7819) (-87.4182, 25.6234) (-87.3833, 25.5555) knots 0 0 0 1 2 2 2
  spline S128 degree 2 poles (-87.3833, 25.5555) (-87.3544, 25.4958) (-87.2248, 25.4361) (-87.1136, 25.4361) knots 0 0 0 1 2 2 2
  spline S129 degree 2 poles (-87.1136, 25.4361) (-87.0354, 25.4361) (-86.8893, 25.4834) (-86.8563, 25.4978) knots 0 0 0 1 2 2 2
  line L117 (-86.8563, 25.4978) -> (-86.8378, 25.4978)
  line L118 (-86.8378, 25.4978) -> (-86.8378, 25.2097)
  spline S130 degree 2 poles (-86.8378, 25.2097) (-86.9284, 25.185) (-87.1136, 25.1562) (-87.1939, 25.1562) knots 0 0 0 1 2 2 2
  spline S131 degree 2 poles (-85.0347, 26.1462) (-85.0347, 25.6646) (-85.4978, 25.1397) (-85.8848, 25.1397) knots 0 0 0 1 2 2 2
  spline S132 degree 2 poles (-85.8848, 25.1397) (-86.282, 25.1397) (-86.7369, 25.681) (-86.7369, 26.1462) knots 0 0 0 1 2 2 2
  spline S133 degree 2 poles (-86.7369, 26.1462) (-86.7369, 26.6238) (-86.2676, 27.1528) (-85.8848, 27.1528) knots 0 0 0 1 2 2 2
  spline S134 degree 2 poles (-85.8848, 27.1528) (-85.4978, 27.1528) (-85.0347, 26.6258) (-85.0347, 26.1462) knots 0 0 0 1 2 2 2
  spline S135 degree 2 poles (-85.3661, 26.1462) (-85.3661, 26.5167) (-85.6357, 26.8769) (-85.8848, 26.8769) knots 0 0 0 1 2 2 2
  spline S136 degree 2 poles (-85.8848, 26.8769) (-86.1338, 26.8769) (-86.4055, 26.5167) (-86.4055, 26.1462) knots 0 0 0 1 2 2 2
  spline S137 degree 2 poles (-86.4055, 26.1462) (-86.4055, 25.786) (-86.1338, 25.4155) (-85.8848, 25.4155) knots 0 0 0 1 2 2 2
  spline S138 degree 2 poles (-85.8848, 25.4155) (-85.6378, 25.4155) (-85.3661, 25.7798) (-85.3661, 26.1462) knots 0 0 0 1 2 2 2
  spline S139 degree 2 poles (-83.1389, 26.1462) (-83.1389, 25.6646) (-83.6021, 25.1397) (-83.989, 25.1397) knots 0 0 0 1 2 2 2
  spline S140 degree 2 poles (-83.989, 25.1397) (-84.3863, 25.1397) (-84.8412, 25.681) (-84.8412, 26.1462) knots 0 0 0 1 2 2 2
  spline S141 degree 2 poles (-84.8412, 26.1462) (-84.8412, 26.6238) (-84.3719, 27.1528) (-83.989, 27.1528) knots 0 0 0 1 2 2 2
  spline S142 degree 2 poles (-83.989, 27.1528) (-83.6021, 27.1528) (-83.1389, 26.6258) (-83.1389, 26.1462) knots 0 0 0 1 2 2 2
  spline S143 degree 2 poles (-83.4703, 26.1462) (-83.4703, 26.5167) (-83.74, 26.8769) (-83.989, 26.8769) knots 0 0 0 1 2 2 2
  spline S144 degree 2 poles (-83.989, 26.8769) (-84.2381, 26.8769) (-84.5098, 26.5167) (-84.5098, 26.1462) knots 0 0 0 1 2 2 2
  spline S145 degree 2 poles (-84.5098, 26.1462) (-84.5098, 25.786) (-84.2381, 25.4155) (-83.989, 25.4155) knots 0 0 0 1 2 2 2
  spline S146 degree 2 poles (-83.989, 25.4155) (-83.742, 25.4155) (-83.4703, 25.7798) (-83.4703, 26.1462) knots 0 0 0 1 2 2 2
  spline S147 degree 2 poles (-80.1214, 26.1771) (-80.1214, 25.7099) (-80.5742, 25.1397) (-80.9159, 25.1397) knots 0 0 0 1 2 2 2
  spline S148 degree 2 poles (-80.9159, 25.1397) (-81.0703, 25.1397) (-81.2905, 25.2159) (-81.3976, 25.2817) knots 0 0 0 1 2 2 2
  line L119 (-81.3976, 25.2817) -> (-81.4182, 25.1932)
  line L120 (-81.4182, 25.1932) -> (-81.7187, 25.1932)
  line L121 (-81.7187, 25.1932) -> (-81.7187, 27.8464)
  line L122 (-81.7187, 27.8464) -> (-81.3976, 27.8464)
  line L123 (-81.3976, 27.8464) -> (-81.3976, 26.8996)
  spline S149 degree 2 poles (-81.3976, 26.8996) (-81.2761, 27.0087) (-80.9941, 27.1528) (-80.8151, 27.1528) knots 0 0 0 1 2 2 2
  spline S150 degree 2 poles (-80.8151, 27.1528) (-80.4919, 27.1528) (-80.1214, 26.6361) (-80.1214, 26.1771) knots 0 0 0 1 2 2 2
  spline S151 degree 2 poles (-80.4528, 26.1524) (-80.4528, 26.4941) (-80.6607, 26.8481) (-80.8912, 26.8481) knots 0 0 0 1 2 2 2
  spline S152 degree 2 poles (-80.8912, 26.8481) (-81.0209, 26.8481) (-81.2885, 26.7246) (-81.3976, 26.6299) knots 0 0 0 1 2 2 2
  line L124 (-81.3976, 26.6299) -> (-81.3976, 25.537)
  spline S153 degree 2 poles (-81.3976, 25.537) (-81.2761, 25.4773) (-81.0888, 25.4279) (-80.9777, 25.4279) knots 0 0 0 1 2 2 2
  spline S154 degree 2 poles (-80.9777, 25.4279) (-80.7327, 25.4279) (-80.4528, 25.7757) (-80.4528, 26.1524) knots 0 0 0 1 2 2 2
  line L125 (-79.4607, 25.1932) -> (-79.7818, 25.1932)
  line L126 (-79.7818, 25.1932) -> (-79.7818, 27.0992)
  line L127 (-79.7818, 27.0992) -> (-79.4607, 27.0992)
  line L128 (-79.4607, 27.0992) -> (-79.4607, 25.1932)
  line L129 (-79.438, 27.4162) -> (-79.8024, 27.4162)
  line L130 (-79.8024, 27.4162) -> (-79.8024, 27.7497)
  line L131 (-79.8024, 27.7497) -> (-79.438, 27.7497)
  line L132 (-79.438, 27.7497) -> (-79.438, 27.4162)
  spline S155 degree 2 poles (-78.9214, 24.8886) (-78.8885, 24.8742) (-78.7629, 24.8289) (-78.6826, 24.8104) knots 0 0 0 1 2 2 2
  spline S156 degree 2 poles (-78.6826, 24.8104) (-78.5941, 24.7877) (-78.4439, 24.761) (-78.3553, 24.761) knots 0 0 0 1 2 2 2
  spline S157 degree 2 poles (-78.3553, 24.761) (-78.2071, 24.761) (-78.0013, 24.8392) (-77.9437, 24.9092) knots 0 0 0 1 2 2 2
  spline S158 degree 2 poles (-77.9437, 24.9092) (-77.8881, 24.9791) (-77.8449, 25.1623) (-77.8449, 25.2797) knots 0 0 0 1 2 2 2
  line L133 (-77.8449, 25.2797) -> (-77.8449, 25.4464)
  spline S159 degree 2 poles (-77.8449, 25.4464) (-77.9746, 25.3332) (-78.2236, 25.2261) (-78.4109, 25.2261) knots 0 0 0 1 2 2 2
  spline S160 degree 2 poles (-78.4109, 25.2261) (-78.7361, 25.2261) (-79.1211, 25.7099) (-79.1211, 26.1647) knots 0 0 0 1 2 2 2
  spline S161 degree 2 poles (-79.1211, 26.1647) (-79.1211, 26.4015) (-78.9873, 26.7678) (-78.8761, 26.8975) knots 0 0 0 1 2 2 2
  spline S162 degree 2 poles (-78.8761, 26.8975) (-78.7691, 27.019) (-78.4747, 27.1528) (-78.3183, 27.1528) knots 0 0 0 1 2 2 2
  spline S163 degree 2 poles (-78.3183, 27.1528) (-78.1701, 27.1528) (-77.954, 27.0828) (-77.8449, 27.019) knots 0 0 0 1 2 2 2
  line L134 (-77.8449, 27.019) -> (-77.8264, 27.0992)
  line L135 (-77.8264, 27.0992) -> (-77.5238, 27.0992)
  line L136 (-77.5238, 27.0992) -> (-77.5238, 25.4114)
  spline S164 degree 2 poles (-77.5238, 25.4114) (-77.5238, 24.9256) (-77.9457, 24.4728) (-78.38, 24.4728) knots 0 0 0 1 2 2 2
  spline S165 degree 2 poles (-78.38, 24.4728) (-78.52, 24.4728) (-78.8123, 24.5181) (-78.9379, 24.5551) knots 0 0 0 1 2 2 2
  line L137 (-78.9379, 24.5551) -> (-78.9379, 24.8886)
  line L138 (-78.9379, 24.8886) -> (-78.9214, 24.8886)
  line L139 (-77.8449, 25.7099) -> (-77.8449, 26.7576)
  spline S166 degree 2 poles (-77.8449, 26.7576) (-77.9643, 26.8152) (-78.166, 26.8646) (-78.2668, 26.8646) knots 0 0 0 1 2 2 2
  spline S167 degree 2 poles (-78.2668, 26.8646) (-78.5097, 26.8646) (-78.7897, 26.5064) (-78.7897, 26.1709) knots 0 0 0 1 2 2 2
  spline S168 degree 2 poles (-78.7897, 26.1709) (-78.7897, 25.8539) (-78.5776, 25.5225) (-78.3389, 25.5225) knots 0 0 0 1 2 2 2
  spline S169 degree 2 poles (-78.3389, 25.5225) (-78.2133, 25.5225) (-77.9499, 25.6213) (-77.8449, 25.7099) knots 0 0 0 1 2 2 2
  line L140 (-94.1429, 21.9683) -> (-95.1041, 21.9683)
  line L141 (-95.1041, 21.9683) -> (-95.1041, 22.277)
  line L142 (-95.1041, 22.277) -> (-94.1429, 22.277)
  line L143 (-94.1429, 22.277) -> (-94.1429, 21.9683)
  spline S170 degree 2 poles (-93.0252, 20.9659) (-93.301, 20.9659) (-93.688, 21.0812) (-93.8588, 21.1635) knots 0 0 0 1 2 2 2
  line L144 (-93.8588, 21.1635) -> (-93.8588, 21.5875)
  line L145 (-93.8588, 21.5875) -> (-93.8341, 21.5875)
  spline S171 degree 2 poles (-93.8341, 21.5875) (-93.6674, 21.4311) (-93.2454, 21.2582) (-93.0499, 21.2582) knots 0 0 0 1 2 2 2
  spline S172 degree 2 poles (-93.0499, 21.2582) (-92.7699, 21.2582) (-92.4838, 21.4908) (-92.4838, 21.6822) knots 0 0 0 1 2 2 2
  spline S173 degree 2 poles (-92.4838, 21.6822) (-92.4838, 21.8345) (-92.6341, 22.0239) (-92.7967, 22.0712) knots 0 0 0 1 2 2 2
  spline S174 degree 2 poles (-92.7967, 22.0712) (-92.914, 22.1041) (-93.1096, 22.1494) (-93.2557, 22.1865) knots 0 0 0 1 2 2 2
  spline S175 degree 2 poles (-93.2557, 22.1865) (-93.3875, 22.2215) (-93.5953, 22.3265) (-93.6756, 22.4108) knots 0 0 0 1 2 2 2
  spline S176 degree 2 poles (-93.6756, 22.4108) (-93.7538, 22.4952) (-93.8403, 22.7217) (-93.8403, 22.8699) knots 0 0 0 1 2 2 2
  spline S177 degree 2 poles (-93.8403, 22.8699) (-93.8403, 23.1786) (-93.3586, 23.5965) (-92.9861, 23.5965) knots 0 0 0 1 2 2 2
  spline S178 degree 2 poles (-92.9861, 23.5965) (-92.772, 23.5965) (-92.3933, 23.5121) (-92.2307, 23.4318) knots 0 0 0 1 2 2 2
  line L146 (-92.2307, 23.4318) -> (-92.2307, 23.0283)
  line L147 (-92.2307, 23.0283) -> (-92.2554, 23.0283)
  spline S179 degree 2 poles (-92.2554, 23.0283) (-92.3768, 23.1395) (-92.7555, 23.3042) (-92.9634, 23.3042) knots 0 0 0 1 2 2 2
  spline S180 degree 2 poles (-92.9634, 23.3042) (-93.1981, 23.3042) (-93.4883, 23.0839) (-93.4883, 22.9048) knots 0 0 0 1 2 2 2
  spline S181 degree 2 poles (-93.4883, 22.9048) (-93.4883, 22.7443) (-93.3175, 22.5529) (-93.1569, 22.5096) knots 0 0 0 1 2 2 2
  spline S182 degree 2 poles (-93.1569, 22.5096) (-93.0499, 22.4808) (-92.7391, 22.4067) (-92.6362, 22.3759) knots 0 0 0 1 2 2 2
  spline S183 degree 2 poles (-92.6362, 22.3759) (-92.3747, 22.2956) (-92.1319, 21.9724) (-92.1319, 21.7357) knots 0 0 0 1 2 2 2
  spline S184 degree 2 poles (-92.1319, 21.7357) (-92.1319, 21.5854) (-92.2533, 21.2973) (-92.3624, 21.1964) knots 0 0 0 1 2 2 2
  spline S185 degree 2 poles (-92.3624, 21.1964) (-92.4838, 21.0853) (-92.7926, 20.9659) (-93.0252, 20.9659) knots 0 0 0 1 2 2 2
  spline S186 degree 2 poles (-90.7507, 21.2129) (-90.7898, 21.1841) (-90.9216, 21.0812) (-90.9833, 21.0503) knots 0 0 0 1 2 2 2
  spline S187 degree 2 poles (-90.9833, 21.0503) (-91.0677, 21.005) (-91.2262, 20.9576) (-91.3703, 20.9576) knots 0 0 0 1 2 2 2
  spline S188 degree 2 poles (-91.3703, 20.9576) (-91.4876, 20.9576) (-91.6996, 21.0462) (-91.7799, 21.1264) knots 0 0 0 1 2 2 2
  spline S189 degree 2 poles (-91.7799, 21.1264) (-91.856, 21.2047) (-91.9487, 21.4352) (-91.9487, 21.5628) knots 0 0 0 1 2 2 2
  spline S190 degree 2 poles (-91.9487, 21.5628) (-91.9487, 21.7604) (-91.7819, 22.0403) (-91.6008, 22.1206) knots 0 0 0 1 2 2 2
  spline S191 degree 2 poles (-91.6008, 22.1206) (-91.4403, 22.1947) (-91.0039, 22.2503) (-90.7507, 22.2647) knots 0 0 0 1 2 2 2
  line L148 (-90.7507, 22.2647) -> (-90.7507, 22.3265)
  spline S192 degree 2 poles (-90.7507, 22.3265) (-90.7507, 22.4376) (-90.8186, 22.5755) (-90.8804, 22.6146) knots 0 0 0 1 2 2 2
  spline S193 degree 2 poles (-90.8804, 22.6146) (-90.9421, 22.6537) (-91.1192, 22.6784) (-91.2138, 22.6784) knots 0 0 0 1 2 2 2
  spline S194 degree 2 poles (-91.2138, 22.6784) (-91.325, 22.6784) (-91.6255, 22.6126) (-91.7758, 22.5488) knots 0 0 0 1 2 2 2
  line L149 (-91.7758, 22.5488) -> (-91.7943, 22.5488)
  line L150 (-91.7943, 22.5488) -> (-91.7943, 22.876)
  spline S195 degree 2 poles (-91.7943, 22.876) (-91.7058, 22.9007) (-91.3744, 22.9625) (-91.2118, 22.9625) knots 0 0 0 1 2 2 2
  spline S196 degree 2 poles (-91.2118, 22.9625) (-91.0142, 22.9625) (-90.7445, 22.9007) (-90.6375, 22.8205) knots 0 0 0 1 2 2 2
  spline S197 degree 2 poles (-90.6375, 22.8205) (-90.5325, 22.7422) (-90.4296, 22.4932) (-90.4296, 22.3141) knots 0 0 0 1 2 2 2
  line L151 (-90.4296, 22.3141) -> (-90.4296, 21.0112)
  line L152 (-90.4296, 21.0112) -> (-90.7507, 21.0112)
  line L153 (-90.7507, 21.0112) -> (-90.7507, 21.2129)
  line L154 (-90.7507, 21.4805) -> (-90.7507, 22.0095)
  spline S198 degree 2 poles (-90.7507, 22.0095) (-90.866, 21.9992) (-91.2138, 21.9642) (-91.3229, 21.9312) knots 0 0 0 1 2 2 2
  spline S199 degree 2 poles (-91.3229, 21.9312) (-91.4505, 21.8921) (-91.6173, 21.7295) (-91.6173, 21.5854) knots 0 0 0 1 2 2 2
  spline S200 degree 2 poles (-91.6173, 21.5854) (-91.6173, 21.4208) (-91.432, 21.2541) (-91.255, 21.2541) knots 0 0 0 1 2 2 2
  spline S201 degree 2 poles (-91.255, 21.2541) (-91.1047, 21.2541) (-90.8577, 21.3837) (-90.7507, 21.4805) knots 0 0 0 1 2 2 2
  line L155 (-89.6516, 21.0112) -> (-89.9727, 21.0112)
  line L156 (-89.9727, 21.0112) -> (-89.9727, 22.9172)
  line L157 (-89.9727, 22.9172) -> (-89.6516, 22.9172)
  line L158 (-89.6516, 22.9172) -> (-89.6516, 21.0112)
  line L159 (-89.6289, 23.2342) -> (-89.9932, 23.2342)
  line L160 (-89.9932, 23.2342) -> (-89.9932, 23.5676)
  line L161 (-89.9932, 23.5676) -> (-89.6289, 23.5676)
  line L162 (-89.6289, 23.5676) -> (-89.6289, 23.2342)
  line L163 (-88.3383, 21.0112) -> (-87.4821, 23.5512)
  line L164 (-87.4821, 23.5512) -> (-87.0663, 23.5512)
  line L165 (-87.0663, 23.5512) -> (-86.21, 21.0112)
  line L166 (-86.21, 21.0112) -> (-86.5661, 21.0112)
  line L167 (-86.5661, 21.0112) -> (-86.7966, 21.7213)
  line L168 (-86.7966, 21.7213) -> (-87.7661, 21.7213)
  line L169 (-87.7661, 21.7213) -> (-87.9966, 21.0112)
  line L170 (-87.9966, 21.0112) -> (-88.3383, 21.0112)
  line L171 (-86.8893, 22.0095) -> (-87.2824, 23.2054)
  line L172 (-87.2824, 23.2054) -> (-87.6735, 22.0095)
  line L173 (-87.6735, 22.0095) -> (-86.8893, 22.0095)
  point P0 (0, 0)
  constraints: 2 other
extrude "Extrusion2" cut sketch "Sketch3" against normal blind 0.2
body "Solid1"
